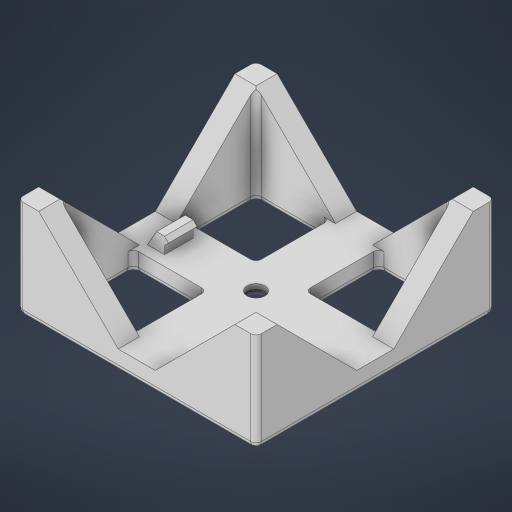
# Autodesk Inventor part: CalibrationBlock
Saved by Autodesk Inventor 2023 (Build 270158000, 158)
## iProperties
Created: 2022-12-27
Part Number: CalibrationBlock
Material: Generic
Document SubType Name: Modeling
Designer: jevan
Density: 1 g/cm^3
Appearance: Default
Author: jevan
Autodesk Inventor part; units mm, degrees
ref_plane "YZ Plane" through (0, 0, 0) normal (1, 0, 0) x (0, 1, 0)
ref_plane "XZ Plane" through (0, 0, 0) normal (0, 1, 0) x (-1, 0, 0)
ref_plane "XY Plane" through (0, 0, 0) normal (0, 0, 1) x (1, 0, 0)
sketch "Sketch1" plane through (0, 0, 0) normal (0, 0, 1) x (1, 0, 0)
  circle A0 centre (0, 0) radius 7.3
  circle A1 centre (0, 0) radius 3.375
  line L0 (18.1665, 0) -> (27.6873, 16.4907)
  line L1 (27.6873, 16.4907) -> (0, 32.476)
  line L2 (0, 32.476) -> (-28.125, 16.238)
  line L3 (-28.125, 16.238) -> (-28.125, -16.238)
  line L4 (-28.125, -16.238) -> (0, -32.476)
  line L5 (0, -32.476) -> (27.6873, -16.4907)
  line L6 (27.6873, -16.4907) -> (18.1665, 0)
  line L7 (0, 0) -> (0, 32.476)
  line L8 (0, 0) -> (18.1665, 0)
  line L9 (-45, -45) -> (45, -45)
  line L10 (45, -45) -> (45, 45)
  line L11 (45, 45) -> (-45, 45)
  line L12 (-45, 45) -> (-45, -45)
  line L13 (21.6306, 0) -> (31.7854, -17.5887)
  line L14 (31.7854, -17.5887) -> (0, -35.9401)
  line L15 (0, -35.9401) -> (-31.125, -17.97)
  line L16 (-31.125, -17.97) -> (-31.125, 17.97)
  line L17 (-31.125, 17.97) -> (0, 35.9401)
  line L18 (0, 35.9401) -> (31.7854, 17.5887)
  line L19 (31.7854, 17.5887) -> (21.6306, 0)
  line L20 (0, -35.9401) -> (0, -45)
  line L21 (0, 35.9401) -> (0, 45)
  line L22 (0, 0) -> (-45, 0)
  line L23 (0, 0) -> (45, 0)
  line L24 (-7.7942, 27.976) -> (-9.2942, 30.574)
  line L25 (7.7942, 27.976) -> (9.2942, 30.574)
  line L26 (-7.7942, -27.976) -> (-9.2942, -30.574)
  line L27 (7.7942, -27.976) -> (9.2942, -30.574)
  line L28 (-45, -45) -> (-37, -45)
  line L29 (-37, -45) -> (-37, -37)
  line L30 (-37, -37) -> (-45, -37)
  line L31 (-45, -37) -> (-45, -45)
  line L32 (-45, 45) -> (-37, 45)
  line L33 (-37, 45) -> (-37, 37)
  line L34 (-37, 37) -> (-45, 37)
  line L35 (-45, 37) -> (-45, 45)
  line L36 (45, 45) -> (37, 45)
  line L37 (37, 45) -> (37, 37)
  line L38 (37, 37) -> (45, 37)
  line L39 (45, 37) -> (45, 45)
  line L40 (45, -45) -> (37, -45)
  line L41 (37, -45) -> (37, -37)
  line L42 (37, -37) -> (45, -37)
  line L43 (45, -37) -> (45, -45)
  line L44 (-6.473, -3.375) -> (6.473, -3.375)
  line L45 (6.473, 3.375) -> (-6.473, 3.375)
  line L46 (3.375, -3.375) -> (3.375, 3.375)
  line L47 (-3.375, -3.375) -> (-3.375, 3.375)
  line L48 (9.2942, 45) -> (9.2942, -45)
  line L49 (-9.2942, 45) -> (-9.2942, -45)
  line L50 (26.1306, 7.7942) -> (23.5325, 9.2942)
  line L51 (37, 9.2942) -> (-37, 9.2942)
  line L52 (37, -9.2942) -> (-37, -9.2942)
  line L53 (-37, 37) -> (37, 37)
  line L54 (37, 37) -> (37, -37)
  line L55 (37, -37) -> (-37, -37)
  line L56 (-37, -37) -> (-37, 37)
  line L57 (18.5129, 0.2) -> (28.2337, -16.6371)
  line L58 (28.2337, -16.6371) -> (0, -32.9378)
  line L59 (0, -32.9378) -> (-28.525, -16.4689)
  line L60 (-28.525, -16.4689) -> (-28.525, 16.4689)
  line L61 (-28.525, 16.4689) -> (0, 32.9378)
  line L62 (18.5129, -0.2) -> (28.2337, 16.6371)
  line L63 (28.2337, 16.6371) -> (-2.6, 34.4389)
  point P0 (37, -45)
  point P1 (37, 45)
  point P2 (-37, 45)
  point P3 (-45, -37)
  point P4 (-3.375, 0)
  point P5 (3.375, 0)
  point P6 (-3.375, 0)
  point P7 (0, 3.375)
  point P8 (0, -3.375)
  point P9 (3.375, 0)
  point P10 (-28.125, 9.2942)
  point P11 (23.5325, -9.2942)
  point P12 (-28.125, -9.2942)
  point P13 (-9.2942, 37)
  point P14 (-9.2942, 9.2942)
  point P15 (9.2942, 37)
  point P16 (9.2942, 9.2942)
  point P17 (9.2942, -9.2942)
  point P18 (9.2942, -37)
  point P19 (-9.2942, -37)
  point P20 (-9.2942, -9.2942)
  point P21 (-9.2942, -27.1099)
  point P22 (9.2942, -27.1099)
  point P23 (-9.2942, 27.1099)
  point P24 (9.2942, 27.1099)
  point P25 (9.2942, 27.5718)
  point P26 (-9.2942, 27.5718)
  point P27 (9.2942, -27.5718)
  point P28 (-9.2942, -27.5718)
  dimension "d3" = 14.6
  dimension "d4" = 6.75
  dimension "d11" = 56.25
  dimension "d12" = 56.25
  dimension "d13" = 31.9706
  dimension "d14" = 32.4759
  dimension "d15" = 32.4759
  dimension "d16" = 3
  dimension "d17" = 3
  dimension "d18" = 3
  dimension "d19" = 3
  dimension "d20" = 9
  dimension "d25" = 8
  dimension "d26" = 8
  dimension "d27" = 8
  dimension "d28" = 8
  dimension "d29" = 8
  dimension "d30" = 8
  dimension "d31" = 8
  dimension "d32" = 8
  dimension "d41" = 90
  dimension "d42" = 90
  dimension "d48" = 9
  dimension "d61" = 0.4
  dimension "d62" = 0.4
  dimension "d63" = 0.4
  dimension "d64" = 0.4
  constraints: 128 end point, 23 point on line, 16 perpendicular, 11 parallel, 10 symmetric about line, 6 equal length, 6 horizontal, 4 midpoint, 4 point on circle, 4 tangent, 3 coincident, 2 centre point, 1 vertical, 7 other
  measures "d3" diameter of A0
  measures "d4" diameter of A1
  measures "d11" distance between parallel lines of L1 L4
  measures "d12" distance between parallel lines of L5 L2
  measures "d13" distance of L0.end L2.start
  measures "d14" distance of L2.end L4.start
  measures "d15" distance of L7.start L2.start
  measures "d16" distance between parallel lines of L4 L15
  measures "d17" distance between parallel lines of L1 L18
  measures "d18" distance between parallel lines of L2 L17
  measures "d19" distance between parallel lines of L19 L0
  measures "d20" distance from line of L2.start L24
  measures "d25" distance of L30.end L29.end
  measures "d26" distance of L29.end L28.end
  measures "d27" distance of L33.end L34.end
  measures "d28" distance of L32.end L33.end
  measures "d29" distance of L38.end L37.end
  measures "d30" distance of L37.end L36.end
  measures "d31" distance of L41.end L42.end
  measures "d32" distance of L40.end L41.end
  measures "d41" distance between parallel lines of L9 L11
  measures "d42" distance between parallel lines of L12 L10
  measures "d48" distance from line of L13.start L50
  measures "d61" distance between parallel lines of L4 L59
  measures "d62" distance between parallel lines of L0 L62
  measures "d63" distance between parallel lines of L61 L2
  measures "d64" distance between parallel lines of L63 L1
extrude "Extrusion2" add sketch "Sketch1" against normal blind 5.6 contours L8 L48 L52 L49 L22 A0 | A0 L7 L51 L48 L8 | L48 L51 L0 L8 | L8 L6 L52 L48 | A0 L22 L49 L51 L7 | L23 L57 L52 L6 | L0 L50 L62 L23 | L51 L7 L1 L48 | L48 L5 L4 L49 L52 | L51 L49 L2 L7 | L51 L62 L50 | L62 L50 L19 L23 | L23 L13 L52 L57 | L1 L25 L63 L48 | L48 L58 L27 L5 | L52 L3 L22 L49 | L2 L24 L61 L63 L25 L1 | L49 L22 L3 L51 | L62 L51 L19 L50 | L23 L54 L52 L13 | L19 L51 L54 L23 | L63 L25 L48 | L27 L58 L59 L26 L4 L5 | L48 L27 L58 | L4 L26 L59 L49 | L52 L60 L22 L3 | L2 L49 L61 L24 | L3 L22 L60 L51 | L54 L38 L10 L23 | L23 L10 L42 L54 | L63 L17 L18 L25 | L18 L21 L53 L48 | L27 L14 L15 L26 L59 L58 | L48 L55 L20 L14 | L59 L26 L49 | L52 L16 L22 L60 | L61 L49 L24 | L24 L17 L63 L61 | L60 L22 L16 L51 | L17 L49 L53 L21 | L53 L21 L11 L48 | L48 L11 L37 L53 | L20 L55 L49 L15 | L55 L41 L9 L48 | L48 L9 L20 L55 | L52 L56 L22 L16 | L16 L22 L56 L51 | L37 L11 L10 L38 | L42 L10 L9 L41 | L53 L49 L11 L21 | L20 L9 L49 L55 | L49 L9 L29 L55 | L56 L30 L12 L22 | L53 L33 L11 L49 | L56 L22 L12 L34 | L29 L9 L12 L30 | L34 L12 L11 L33
extrude "Extrusion3" add sketch "Sketch1" along normal blind 30 contours L54 L38 L10 L23 | L23 L10 L42 L54 | L53 L21 L11 L48 | L48 L11 L37 L53 | L55 L41 L9 L48 | L48 L9 L20 L55 | L37 L11 L10 L38 | L42 L10 L9 L41 | L53 L49 L11 L21 | L20 L9 L49 L55 | L49 L9 L29 L55 | L56 L30 L12 L22 | L53 L33 L11 L49 | L56 L22 L12 L34 | L29 L9 L12 L30 | L34 L12 L11 L33
extrude "Extrusion4" add sketch "Sketch1" against normal blind 0.9 contours L45 L7 A0 | A0 L44 | L7 L45 A0
extrude "Extrusion5" add sketch "Sketch1" against normal blind 0.6 contours L8 L46 L45 A0 | A0 L44 L46 L8 | A0 L22 L47 L44 | L45 L47 L22 A0
extrude "Extrusion6" add sketch "Sketch1" against normal blind 0.3 contours L46 L44 A1 | A1 L45 L46 | A1 L47 L45 | L44 L47 A1
sketch "Sketch3" plane through (45, -45, -5.6) normal (1, 0, 0) x (0, 0, -1)
  line L0 (0, 8) -> (-35.6, 8) projected
  line L1 (-35.6, 8) -> (-5.6, 38)
  line L2 (-5.6, 35.7058) -> (-5.6, 54.2942) projected
  line L3 (0, 52.3) -> (0, 37.7) projected
  line L4 (0, 45) -> (-35.6, 45)
  line L5 (-35.6, 82) -> (-35.6, 8) projected
  line L6 (-5.6, 54.2942) -> (-5.6, 35.7058) projected
  line L7 (-33.4787, 5.8787) -> (-3.4787, 35.8787)
  line L8 (0, 82) -> (-35.6, 82)
  line L9 (-35.6, 82) -> (-5.6, 52)
  line L10 (-5.6, 82) -> (-5.6, 54.2942)
  line L11 (-33.4787, 84.1213) -> (-3.4787, 54.1213)
  line L12 (-5.6, 82) -> (-5.6, 8) projected
  line L13 (-5.6, 14.426) -> (-5.6, 8)
  point P0 (-5.6, 45)
  point P1 (-5.6, 75.574)
  point P2 (-31.3574, 82)
  point P3 (-5.6, 56.2426)
  point P4 (-5.6, 52)
  point P5 (-5, 33.7574)
  point P6 (-31.3574, 8)
  point P7 (-5.6, 33.7574)
  dimension "d49" = 45
  dimension "d50" = 3
  constraints: 16 end point, 4 symmetric about line, 3 point on line, 2 midpoint, 1 collinear, 1 parallel
  measures "d49" angle of L6 L1
  measures "d50" distance between parallel lines of L1 L7
extrude "Extrusion8" cut sketch "Sketch3" against normal through all contours L5 L4 L2 L1 | L5 L9 L2 L4
sketch "Sketch4" plane through (-45, 45, -5.6) normal (0, 1, 0) x (1, 0, 0)
  line L0 (82, 0) -> (82, -35.6) projected
  line L1 (82, -35.6) -> (52, -5.6)
  line L2 (54.2942, -5.6) -> (82, -5.6) projected
  line L3 (35.7058, -5.6) -> (54.2942, -5.6) projected
  line L4 (52, -5.6) -> (54.2942, -5.6)
  line L5 (54.2942, -5.6) -> (52, -5.6)
  line L6 (82, -30.7574) -> (82, -5.6) projected
  line L7 (82, -5.6) -> (82, 0) projected
  line L8 (82, -30.7574) -> (82, -5.6)
  line L9 (45, -5.6) -> (45, -35.6)
  line L10 (90, -35.6) -> (0, -35.6) projected
  line L11 (84.1213, -33.4787) -> (54.1213, -3.4787)
  line L12 (8, -30.7574) -> (8, -35.6)
  line L13 (8, -35.6) -> (38, -5.6)
  line L14 (35.7058, -5.6) -> (8, -5.6)
  line L15 (38, -5.6) -> (35.7058, -5.6)
  line L16 (35.7058, -5.6) -> (38, -5.6)
  line L17 (8, -30.7574) -> (8, -5.6)
  line L18 (8, -5.6) -> (8, 0)
  line L19 (8, -30.7574) -> (8, -5.6)
  line L20 (5.8787, -33.4787) -> (35.8787, -3.4787)
  point P0 (-30.7574, 82)
  point P1 (-5, 56.2426)
  point P2 (-5, 52)
  point P3 (-5, 33.7574)
  point P4 (-30.7574, 8)
  point P5 (33.7574, -5.6)
  point P6 (8, -35.6)
  point P7 (56.2426, -5.6)
  dimension "d55" = 45
  dimension "d56" = 3
  constraints: 30 end point, 7 symmetric about line, 3 collinear, 2 point on line, 1 midpoint, 1 parallel, 1 vertical
  measures "d55" angle of L2 L1
  measures "d56" distance between parallel lines of L1 L11
extrude "Extrusion9" cut sketch "Sketch4" against normal through all contours L10 L9 L3 L1 | L10 L13 L3 L9
sketch "Sketch5" plane through (0, 0, 0) normal (0, 0, 1) x (1, 0, 0)
  line L0 (0, 0) -> (-29.125, 0)
  line L1 (-29.125, 0) -> (-29.125, 5.4)
  line L2 (-29.125, 5.4) -> (-32.125, 5.4)
  line L3 (-32.125, 5.4) -> (-32.125, 0)
  line L4 (-32.125, 0) -> (-29.125, 0)
  line L5 (-29.125, 0) -> (-29.125, -5.4)
  line L6 (-29.125, -5.4) -> (-32.125, -5.4)
  line L7 (-32.125, -5.4) -> (-32.125, 0)
  dimension "d65" = 29.125
  dimension "d66" = 5.4
  dimension "d67" = 3
  constraints: 16 end point, 3 perpendicular, 2 symmetric about line, 1 horizontal, 1 vertical
  measures "d65" distance of L0.start L0.end
  measures "d66" distance of L0.end L1.end
  measures "d67" distance between parallel lines of L1 L3
extrude "Extrusion11" add sketch "Sketch5" along normal blind 6
sketch "Sketch6" plane through (-29.125, -5.4, 0) normal (1, 0, 0) x (0, 0, -1)
  line L0 (0, 0) -> (-6, 0) projected
  line L1 (-6, 0) -> (-3, 0)
  line L2 (-3, 0) -> (-3, 10.8)
  line L3 (0, 10.8) -> (-6, 10.8) projected
  line L4 (-6, 10.8) -> (-6, 0) projected
  line L5 (-6, 0) -> (-6, 10.8)
  point P0 (0, 5.4)
  constraints: 6 end point, 2 midpoint, 1 collinear
extrude "Extrusion12" add sketch "Sketch6" along normal blind 1.5
chamfer "Chamfer2" distance 1.5 angle 45 2 edges at (-27.625, 0, 3) (-27.625, 0, 6)
chamfer "Chamfer3" distance 6 angle 30 1 edges at (-32.125, 0, 0) measured on face at (-32.125, 0, 0.5)
move faces "Move1" translate (0, 0, -1.6) faces at (-3.0981, 42.3333, -5.6) (-1.8248, 3.8598, -0.9) (-4.6833, 0, -0.6) (-2.706, 2.706, -0.3) (2.706, 2.706, -0.3) (4.6833, 0, -0.6) (-1.6373, -5.3999, -0.9) (2.706, -2.706, -0.3) (-2.706, -2.706, -0.3)
fillet "Fillet1" radius 2 41 edges at (45, 0, -7.2) (0, 45, -7.2) (45, 45, 11.4) (-45, 45, 11.4) (-45, 0, -7.2) (0, -45, -7.2) (23.1471, -37, -7.2) (37, -23.1471, -7.2) (9.2942, -23.1471, -7.2) (23.1471, -9.2942, -7.2) (23.1471, 9.2942, -7.2) (9.2942, 23.1471, -7.2) (23.1471, 37, -7.2) (37, 23.1471, -7.2) (-23.1471, 9.2942, -7.2) (-9.2942, 23.1471, -7.2) (-37, 23.1471, -7.2) (-23.1471, 37, -7.2) (-37, -23.1471, -7.2) (-23.1471, -37, -7.2) (-9.2942, -23.1471, -7.2) (-23.1471, -9.2942, -7.2) (45, -45, 11.4) (-45, -45, 11.4) (-7.3, 0, -7.2) (-37, -9.2942, -3.6) (-37, -37, 11.4) (-9.2942, -37, -3.6) (-9.2942, -9.2942, -3.6) (9.2942, -9.2942, -3.6) (9.2942, -37, -3.6) (-37, 37, 11.4) (-9.2942, 37, -3.6) (-9.2942, 9.2942, -3.6) (9.2942, 9.2942, -3.6) (9.2942, 37, -3.6) (37, 37, 11.4) (37, -9.2942, -3.6) (37, -37, 11.4) (37, 9.2942, -3.6) (-37, 9.2942, -3.6)
body "Solid1"
